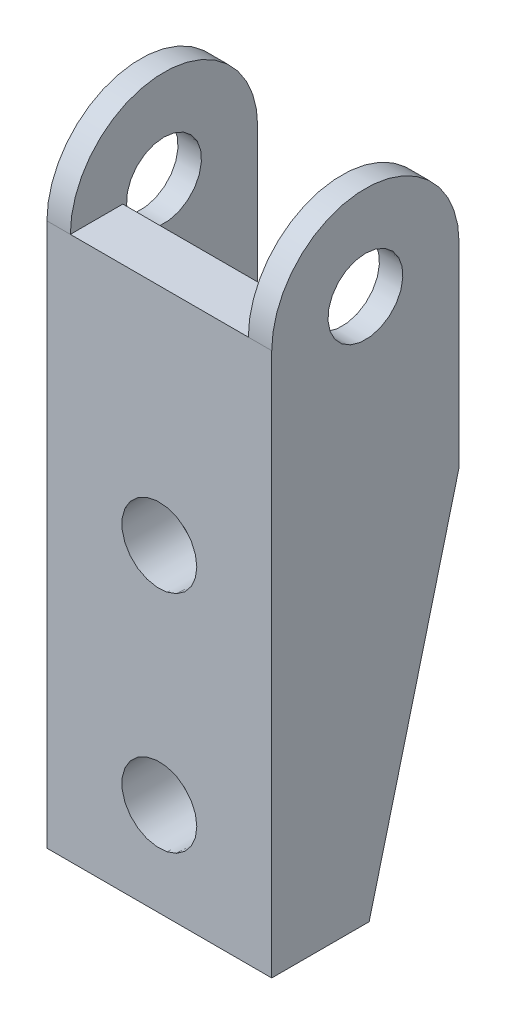
# Autodesk Inventor part: крепленеи кабеля
Saved by Autodesk Inventor 2017 (Build 210142000, 142)
## iProperties
Part Number: крепленеи кабеля
Material: Типовые
Document SubType Name: Modeling
Designer: Max
Mass: 1.38119 g
Surface Area: 17.8037 cm^2
Volume: 1.38119 cm^3
Density: 1 g/cm^3
Appearance: Резина — черная
Author: Max
Autodesk Inventor part; units mm, degrees
ref_plane "YZ Plane" through (0, 0, 0) normal (1, 0, 0) x (0, 1, 0)
ref_plane "XZ Plane" through (0, 0, 0) normal (0, 1, 0) x (-1, 0, 0)
ref_plane "XY Plane" through (0, 0, 0) normal (0, 0, 1) x (1, 0, 0)
sketch "Эскиз1" plane through (0, 0, 0) normal (1, 0, 0) x (0, 1, 0)
  circle A0 centre (0, 0) radius 2
  arc A1 (-4.49, 2.2) -> (0, 5) centre (0, 0) ccw
  line L0 (0, 5) -> (-29, 5)
  line L1 (-29, 5) -> (-29, -0.2)
  line L2 (-29, -0.2) -> (-10.4, -5)
  line L3 (-10.4, -5) -> (0, -5)
  line L4 (-4.49, 2.2) -> (-29, 2.2)
  line L5 (-4.49, 5) -> (0, 5)
  line L6 (-4.49, 5) -> (-29, 5)
  line L7 (-10.4, -5) -> (0, -5)
  line L8 (-4.49, 2.2) -> (0, 2.2)
  line L9 (0, 2.2) -> (0, 5)
  line L10 (0, 5) -> (-4.49, 5)
  dimension "d0" = 4
  dimension "d1" = 10
  dimension "d2" = 34
  dimension "d3" = 5.2
  dimension "d4" = 18.6
  dimension "d5" = 2.8
  dimension "d6" = 10
  constraints: 22 end point, 3 collinear, 3 perpendicular, 3 point on circle, 3 tangent, 2 centre point, 2 coincident, 2 horizontal, 2 point on line, 1 parallel
  measures "d0" diameter of A0
  measures "d1" diameter of A1
  measures "d3" distance of L0.end L1.end
  measures "d4" distance from line of L1 L2.end
  measures "d5" distance between parallel lines of L4 L0
  measures "d6" distance between parallel lines of L0 L3
extrude "Выдавливание1" add sketch "Эскиз1" along normal mid plane 12
extrude "Выдавливание2" cut sketch "Эскиз1" along normal mid plane 9.5 contours L8 L9 A1
extrude "Выдавливание3" cut sketch "Эскиз1" along normal mid plane 9.5 contours A1 L3 L2 L1 L4
sketch "Эскиз2" plane through (-6, -29, 5) normal (0, 0, 1) x (1, 0, 0)
  line L0 (6, 29) -> (6, 0) construction
  line L1 (0, 0) -> (12, 0) construction
  circle A0 centre (6, 5) radius 2
  circle A1 centre (6, 17) radius 2
  dimension "d13" = 4
  dimension "d14" = 4
  dimension "d15" = 12
  dimension "d16" = 5
  constraints: 2 centre point, 2 end point, 2 point on line, 1 midpoint
  measures "d13" diameter of A0
  measures "d14" diameter of A1
  measures "d15" distance of A1.centre A0.centre
  measures "d16" distance from line of L1 A0.centre
extrude "Выдавливание4" cut sketch "Эскиз2" against normal blind 9.5
